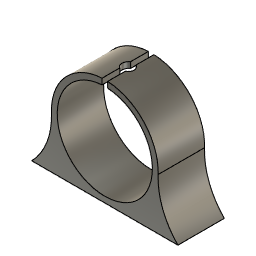
Spar Holes v3 (Autodesk Fusion 360 design; units mm, degrees)
Autodesk Fusion 360 part; units mm, degrees
sketch "Sketch1" plane through (0, 0, 0) normal (0, 1, 0) x (1, 0, 0)
  line L0 (-40.005, 0) -> (40.005, 0)
  line L1 (0, -29.21) -> (0, 0) construction
  line L2 (-1.524, -55.2004) -> (-1.524, -58.3802)
  line L3 (1.524, -55.2004) -> (1.524, -58.3802)
  line L4 (-1.524, -56.7903) -> (1.524, -56.7903) construction
  arc A0 (1.524, -55.2004) -> (-1.524, -55.2004) centre (0, -29.21) ccw
  arc A1 (40.005, 0) -> (29.1884, -28.0872) centre (67.2603, -26.6226) ccw
  arc A2 (-29.1884, -28.0872) -> (-40.005, 0) centre (-67.2603, -26.6226) ccw
  arc A3 (1.524, -58.3802) -> (29.1884, -28.0872) centre (0, -29.21) ccw
  arc A4 (-29.1884, -28.0872) -> (-1.524, -58.3802) centre (0, -29.21) ccw
  dimension "d1" = 52.07
  dimension "d2" = 29.21
  dimension "d3" = 80.01
  dimension "d4" = 58.42
  dimension "d5" = 3.048
  dimension "d7" = 38.1
  constraint horizontal L0
  constraint coincident L1.start A0.centre
  constraint coincident L1.end origin
  constraint perpendicular L0 L1
  constraint midpoint L1.end L0
  constraint concentric A0 A3
  constraint vertical L2
  constraint parallel L2 L3
  constraint midpoint L2 L4.start
  constraint midpoint L3 L4.end
  constraint horizontal L4
  constraint coincident A2.start A3
  constraint tangent A1 A3
  constraint tangent A2 A3
  constraint equal A1 A2
  constraint concentric A3 A4
  measures "d1" diameter of A0
  measures "d2" distance of L1.end L1.start
  measures "d3" distance of L0.start L0.end
  measures "d4" diameter of A3
  measures "d5" distance of L4.start L4.end
  measures "d7" radius of A2
extrude "Extrude1" add sketch "Sketch1" along normal blind 25.4
sketch "Sketch2" plane through (0, 0, 0) normal (0, 0, 1) x (1, 0, 0)
  circle A0 centre (0, 12.7) radius 3.302
  line L0 (-1.524, 25.4) -> (-29.21, 25.4)
  line L1 (-1.524, 0) -> (-29.21, 0)
  line L2 (-5.6643, 25.4) -> (-5.6643, 0) construction
  line L3 (-5.6643, 12.7) -> (0, 12.7) construction
  line L4 (1.524, 0) -> (1.524, 25.4) construction
  line L5 (-1.524, 0) -> (-1.524, 25.4) construction
  line L6 (0, 12.7) -> (0, 14.224) construction
  line L7 (0, 14.224) -> (-1.524, 14.224) construction
  line L8 (0, 14.224) -> (1.524, 14.224) construction
  dimension "d10" = 6.604
  constraint coincident L0 L2.start
  constraint coincident L1 L2.end
  constraint perpendicular L1 L2
  constraint midpoint L2 L3.start
  constraint perpendicular L2 L3
  constraint coincident A0.centre L3.end
  constraint perpendicular L3 L6
  constraint coincident L5 L7.end
  constraint perpendicular L5 L7
  constraint coincident L4 L8.end
  constraint perpendicular L4 L8
  constraint equal L7 L8
  measures "d10" diameter of A0
extrude "Extrude2" cut sketch "Sketch2" along normal blind 65.6387 and the other way blind -9.7561
